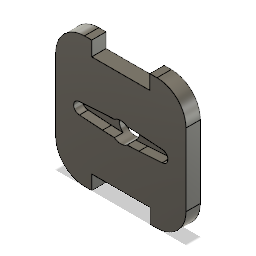
gripper_back (Autodesk Fusion 360 design; units mm, degrees)
Autodesk Fusion 360 part; units mm, degrees
sketch "Sketch2" plane through (0, 0, 0) normal (0, 0, 1) x (1, 0, 0)
  line L0 (-22.5, 22.5) -> (-22.5, -22.5)
  line L1 (22.5, -22.5) -> (22.5, 22.5)
  line L2 (22.5, 22.5) -> (-22.5, -22.5) construction
  line L3 (-22.5, 22.5) -> (22.5, -22.5) construction
  line L4 (10, 22.5) -> (10, 17.5)
  line L5 (-10, 22.5) -> (-10, 17.5)
  line L6 (-10, 17.5) -> (10, 17.5)
  line L7 (22.5, 22.5) -> (10, 22.5)
  line L8 (-10, 22.5) -> (-22.5, 22.5)
  line L9 (-10, -17.5) -> (10, -17.5)
  line L10 (10, -17.5) -> (10, -22.5)
  line L11 (-10, -17.5) -> (-10, -22.5)
  line L12 (-22.5, -22.5) -> (-10, -22.5)
  line L13 (10, -22.5) -> (22.5, -22.5)
  line L14 (-12.5, -22.5) -> (-10, -22.5)
  line L15 (-10, -22.5) -> (-10, -17.5)
  line L16 (10, -22.5) -> (12.5, -22.5)
  line L17 (-12.5, -22.5) -> (-10, -22.5)
  line L18 (-10, -22.5) -> (-10, -17.5)
  line L19 (10, -22.5) -> (12.5, -22.5)
  dimension "d1" = 45
  dimension "d2" = 45
  dimension "d3" = 5
  dimension "d4" = 12.5
  dimension "d5" = 5
  dimension "d6" = 12.5
  dimension "d7" = 35
  constraint perpendicular L0 L7
  constraint parallel L7 L12
  constraint parallel L0 L1
  constraint horizontal L7
  constraint coincident L2 origin
  constraint coincident L3 origin
  constraint perpendicular L4 L7
  constraint coincident L5.start L7
  constraint perpendicular L5 L7
  constraint collinear L7 L8
  constraint coincident L10.end L12
  constraint perpendicular L10 L12
  constraint perpendicular L11 L12
  constraint collinear L12 L13
  measures "d1" distance of L0.end L1.start
  measures "d2" distance of L0.start L0.end
  measures "d3" distance of L4.start L4.end
  measures "d4" distance of L1 L4
  measures "d5" distance of L5.start L5.end
  measures "d6" distance of L0 L5
extrude "Extrude1" add sketch "Sketch2" along normal blind 5
fillet "Fillet1" radius 10 4 edges at (22.5, 22.5, 2.5) (-22.5, 22.5, 2.5) (-22.5, -22.5, 2.5) (22.5, -22.5, 2.5)
sketch "Sketch3" plane through (0, 0, 5) normal (0, 0, 1) x (1, 0, 0)
  arc A0 (12.5, -22.5) -> (22.5, -12.5) centre (12.5, -12.5) ccw
  line L0 (22.5, -12.5) -> (22.5, 12.5)
  arc A1 (22.5, 12.5) -> (12.5, 22.5) centre (12.5, 12.5) ccw
  line L1 (12.5, 22.5) -> (10, 22.5)
  line L2 (10, 22.5) -> (10, 17.5)
  line L3 (10, 17.5) -> (-10, 17.5)
  line L4 (-10, 17.5) -> (-10, 22.5)
  line L5 (-10, 22.5) -> (-12.5, 22.5)
  arc A2 (-12.5, 22.5) -> (-22.5, 12.5) centre (-12.5, 12.5) ccw
  line L6 (-22.5, 12.5) -> (-22.5, -12.5)
  arc A3 (-22.5, -12.5) -> (-12.5, -22.5) centre (-12.5, -12.5) ccw
  line L7 (-12.5, -22.5) -> (-10, -22.5)
  line L8 (-10, -22.5) -> (-10, -17.5)
  line L9 (-10, -17.5) -> (10, -17.5)
  line L10 (10, -17.5) -> (10, -22.5)
  line L11 (10, -22.5) -> (12.5, -22.5)
  circle A4 centre (0, 0) radius 3.5
  dimension "d11" = 7
  constraint coincident A4.centre origin
  measures "d11" diameter of A4
extrude "Extrude2" cut sketch "Sketch3" against normal blind 5 contours A4
sketch "Sketch4" plane through (0, 0, 5) normal (0, 0, 1) x (1, 0, 0)
  circle A0 centre (0, 0) radius 3.5
  arc A1 (12.5, -22.5) -> (22.5, -12.5) centre (12.5, -12.5) ccw
  line L0 (22.5, -12.5) -> (22.5, 12.5)
  arc A2 (22.5, 12.5) -> (12.5, 22.5) centre (12.5, 12.5) ccw
  line L1 (12.5, 22.5) -> (10, 22.5)
  line L2 (10, 22.5) -> (10, 17.5)
  line L3 (10, 17.5) -> (-10, 17.5)
  line L4 (-10, 17.5) -> (-10, 22.5)
  line L5 (-10, 22.5) -> (-12.5, 22.5)
  arc A3 (-12.5, 22.5) -> (-22.5, 12.5) centre (-12.5, 12.5) ccw
  line L6 (-22.5, 12.5) -> (-22.5, -12.5)
  arc A4 (-22.5, -12.5) -> (-12.5, -22.5) centre (-12.5, -12.5) ccw
  line L7 (-12.5, -22.5) -> (-10, -22.5)
  line L8 (-10, -22.5) -> (-10, -17.5)
  line L9 (-10, -17.5) -> (10, -17.5)
  line L10 (10, -17.5) -> (10, -22.5)
  line L11 (10, -22.5) -> (12.5, -22.5)
  ellipse E0 centre (0, 0) end of major axis (16.25, 0) minor radius 2.75
  line L12 (-16.25, 0) -> (16.25, 0)
  line L13 (0, -2.75) -> (0, 2.75)
  circle A5 centre (14.25, 0) radius 2
  line L14 (14.25, 2) -> (6.2681, 2.5372)
  line L15 (14.25, -2) -> (6.2681, -2.5372)
  circle A6 centre (-14.25, 0) radius 2
  line L16 (-14.25, 2) -> (-6.2681, 2.5372)
  line L17 (-14.25, -2) -> (-6.2681, -2.5372)
  dimension "d14" = 32.5
  dimension "d15" = 5.5
  dimension "d16" = 4
  dimension "d17" = 8
  dimension "d18" = 8
  dimension "d19" = 4
  dimension "d20" = 8
  dimension "d21" = 8
  constraint coincident A0.centre E0.centre
  constraint horizontal L12
  constraint coincident E0 L12.start
  constraint coincident E0 L12.end
  constraint coincident E0 L13.start
  constraint coincident E0 L13.end
  constraint coincident L12.end A5
  constraint coincident A5 L14.start
  constraint coincident E0 L14.end
  constraint coincident A5 L15.start
  constraint coincident E0 L15.end
  constraint coincident L12.start A6
  constraint coincident A6 L16.start
  constraint coincident E0 L16.end
  constraint coincident A6 L17.start
  constraint coincident E0 L17.end
  measures "d14" distance of E0
  measures "d16" diameter of A5
  measures "d17" distance of L14.start L14.end
  measures "d18" distance of L15.start L15.end
  measures "d19" diameter of A6
  measures "d20" distance of L16.start L16.end
  measures "d21" distance of L17.start L17.end
extrude "Extrude3" cut sketch "Sketch4" against normal blind 3 contours A0 E0 L12 A5 | A0 E0 L12 A5 | E0 L12 A5 | E0 L12 A5 | A0 E0 L12 A6 | E0 A5 L14 | A0 E0 L12 A6 | E0 A5 L15 | E0 A5 | E0 A5 | E0 A6 L16 | E0 A6 L17 | E0 L12 A6 | E0 L12 A6 | E0 A6 | E0 A6
